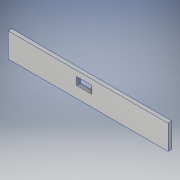
# Autodesk Inventor part: latchplate2
Saved by Autodesk Inventor 2017 (Build 210142000, 142)
## iProperties
Created: 2017-08-11
Part Number: latchplate2
Material: Aluminum 6061
Document SubType Name: Modeling
Designer: Kai
Density: 2.7 g/cm^3
Appearance: Aluminum - Flat
Author: Kai
Autodesk Inventor part; units mm, degrees
ref_plane "YZ Plane" through (0, 0, 0) normal (1, 0, 0) x (0, 1, 0)
ref_plane "XZ Plane" through (0, 0, 0) normal (0, 1, 0) x (-1, 0, 0)
ref_plane "XY Plane" through (0, 0, 0) normal (0, 0, 1) x (1, 0, 0)
sketch "Sketch1" plane through (0, 0, 0) normal (0, 0, 1) x (1, 0, 0)
  line L0 (0, 0) -> (266.7, 0)
  line L1 (266.7, 0) -> (266.7, 40.64)
  line L2 (266.7, 40.64) -> (0, 40.64)
  line L3 (0, 40.64) -> (0, 0)
  line L4 (114.3, 31.75) -> (139.7, 31.75)
  line L5 (139.7, 31.75) -> (139.7, 19.05)
  line L6 (139.7, 19.05) -> (114.3, 19.05)
  line L7 (114.3, 19.05) -> (114.3, 31.75)
  dimension "d0" = 266.7
  dimension "d1" = 40.64
  dimension "d2" = 25.4
  dimension "d3" = 12.7
  dimension "d4" = 19.05
  dimension "d5" = 127
  constraints: 16 end point, 4 parallel, 2 horizontal, 2 perpendicular
  measures "d0" distance of L2.end L1.end
  measures "d1" distance of L1.end L0.end
  measures "d2" distance of L5.end L6.end
  measures "d3" distance of L4.end L5.end
  measures "d4" distance between parallel lines of L6 L0
  measures "d5" distance between parallel lines of L1 L5
extrude "Extrusion1" add sketch "Sketch1" along normal blind 6.35
body "Solid1"
